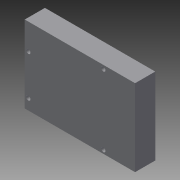
# Autodesk Inventor part: Part8
Saved by Autodesk Inventor 2015 (Build 190159000, 159)
## iProperties
Created: 2015-06-07
Part Number: Part8
Material: Generic
Document SubType Name: Modeling
Designer: Jufo
Density: 1 g/cm^3
Appearance: Default
Author: Jufo
Autodesk Inventor part; units mm, degrees
ref_plane "YZ Plane" through (0, 0, 0) normal (1, 0, 0) x (0, 1, 0)
ref_plane "XZ Plane" through (0, 0, 0) normal (0, 1, 0) x (-1, 0, 0)
ref_plane "XY Plane" through (0, 0, 0) normal (0, 0, 1) x (1, 0, 0)
sketch "Sketch1" plane through (0, 0, 0) normal (0, 1, 0) x (-1, 0, 0)
  line L0 (-32.9824, 25.4864) -> (43.5176, 25.4864)
  line L1 (43.5176, 25.4864) -> (43.5176, -27.9136)
  line L2 (43.5176, -27.9136) -> (-32.9824, -27.9136)
  line L3 (-32.9824, -27.9136) -> (-32.9824, 25.4864)
  circle A0 centre (41.0176, -20.4136) radius 1.5
  circle A1 centre (41.0176, 7.5864) radius 1.5
  circle A2 centre (-10.9824, 22.9864) radius 1.5
  circle A3 centre (-10.9824, -25.4136) radius 1.5
  point P0 (0, 0)
  dimension "d0" = 53.4
  dimension "d2" = 76.5
  dimension "d3" = 3
  dimension "d4" = 3
  dimension "d5" = 3
  dimension "d6" = 3
  dimension "d7" = 2.5
  dimension "d8" = 7.5
  dimension "d9" = 28
  dimension "d10" = 2.5
  dimension "d11" = 52
  dimension "d12" = 2.5
  dimension "d13" = 52
  dimension "d16" = 2.5
  constraints: 8 end point, 4 centre point, 2 parallel, 1 horizontal, 1 perpendicular
  measures "d0" distance of L2.end L0.start
  measures "d2" distance of L0.start L0.end
  measures "d3" diameter of A0
  measures "d4" diameter of A1
  measures "d5" diameter of A2
  measures "d6" diameter of A3
  measures "d7" distance from line of L1 A0.centre
  measures "d8" distance from line of L2 A0.centre
  measures "d9" distance of A0.centre A1.centre
  measures "d10" distance from line of L1 A1.centre
  measures "d11" horizontal distance of A3.centre A0.centre
  measures "d12" distance from line of L0 A2.centre
  measures "d13" horizontal distance of A1.centre A2.centre
  measures "d16" distance from line of L2 A3.centre
extrude "Extrusion1" add sketch "Sketch1" along normal blind 14
body "Solid1"
